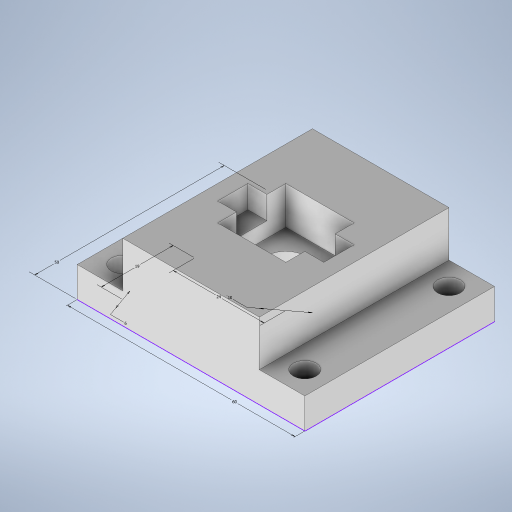
# Autodesk Inventor part: Bartosz_Zukowski_model_nr_7
Saved by Autodesk Inventor 2024 (Build 280153000, 153)
## iProperties
Created: 2024-03-20
Part Number: Bartosz_Zukowski_model_nr_7
Material: Ogólny
Document SubType Name: Modeling
Designer: student156p
Density: 1 g/cm^3
Appearance: Domyślna
Author: student156p
Autodesk Inventor part; units mm, degrees
ref_plane "YZ Plane" through (0, 0, 0) normal (1, 0, 0) x (0, 1, 0)
ref_plane "XZ Plane" through (0, 0, 0) normal (0, 1, 0) x (-1, 0, 0)
ref_plane "XY Plane" through (0, 0, 0) normal (0, 0, 1) x (1, 0, 0)
sketch "podstawa" plane through (0, 0, 0) normal (0, 0, 1) x (1, 0, 0)
  line L0 (-30, -25) -> (30, -25)
  line L1 (30, -25) -> (30, 25)
  line L2 (30, 25) -> (-30, 25)
  line L3 (-30, 25) -> (-30, -25)
  circle A0 centre (0, 0) radius 5
  line L4 (0, 0) -> (24, 0) construction
  line L5 (24, 0) -> (24, 19) construction
  circle A1 centre (24, 19) radius 3
  line L6 (0, 25) -> (0, -25) construction
  circle A2 centre (-24, 19) radius 3
  line L7 (-30, 0) -> (30, 0) construction
  circle A3 centre (24, -19) radius 3
  circle A4 centre (-24, -19) radius 3
  dimension "d0" = 60
  dimension "d1" = 50
  dimension "d9" = 10
  dimension "d26" = 24
  dimension "d27" = 19
  dimension "d28" = 6
  constraints: 16 end point, 5 centre point, 4 midpoint, 3 symmetric about line, 2 coincident, 2 horizontal, 2 parallel, 2 perpendicular, 3 other
  measures "d0" distance of L1.end L2.end
  measures "d1" distance of L0.end L1.end
  measures "d9" diameter of A0
  measures "d26" distance of L4.start L4.end
  measures "d27" distance of L4.end L5.end
  measures "d28" diameter of A1
extrude "Wyciągnięcie proste1" add sketch "podstawa" along normal blind 8 contours L3 L2 L1 L0 | A1 | A2 | A3 | A4
sketch "nakladka" plane through (0, 0, 8) normal (0, 0, 1) x (1, 0, 0)
  line L0 (18, -25) -> (-18, -25)
  line L1 (-18, -25) -> (-18, 25)
  line L2 (-18, 25) -> (18, 25)
  line L3 (18, 25) -> (18, -25)
  line L4 (18, -25) -> (-18, 25) construction
  line L5 (-18, -25) -> (18, 25) construction
  line L6 (-9, -9) -> (9, -9)
  line L7 (9, -9) -> (9, 9)
  line L8 (9, 9) -> (-9, 9)
  line L9 (-9, 9) -> (-9, -9)
  line L10 (-9, -9) -> (9, 9) construction
  line L11 (9, -9) -> (-9, 9) construction
  point P0 (0, 0)
  dimension "d12" = 36
  dimension "d13" = 50
  dimension "d14" = 18
  dimension "d15" = 18
  constraints: 24 end point, 4 midpoint, 4 parallel, 2 horizontal, 2 perpendicular
  measures "d12" distance of L1.end L2.end
  measures "d13" distance of L2.end L0.start
  measures "d14" distance of L7.end L8.end
  measures "d15" distance of L6.end L7.end
extrude "Wyciągnięcie proste2" add sketch "nakladka" along normal blind 12
sketch "srodek_2mm" plane through (0, 0, 8) normal (0, 0, 1) x (1, 0, 0)
  line L0 (-9, -9) -> (9, -9)
  line L1 (9, -9) -> (9, 9)
  line L2 (9, 9) -> (-9, 9)
  line L3 (-9, 9) -> (-9, -9)
  line L4 (-9, -9) -> (9, 9) construction
  line L5 (9, -9) -> (-9, 9) construction
  circle A0 centre (0, 0) radius 5
  constraints: 12 end point, 2 midpoint, 2 parallel, 1 centre point, 1 coincident, 1 horizontal, 1 perpendicular
extrude "Wyciągnięcie proste3" add sketch "srodek_2mm" along normal blind 2
sketch "wyciecie_gora_6mm" plane through (0, 0, 20) normal (0, 0, 1) x (1, 0, 0)
  line L0 (-14, -4) -> (14, -4)
  line L1 (14, -4) -> (14, 4)
  line L2 (14, 4) -> (-14, 4)
  line L3 (-14, 4) -> (-14, -4)
  line L4 (-14, -4) -> (14, 4) construction
  line L5 (14, -4) -> (-14, 4) construction
  point P0 (0, 0)
  dimension "d20" = 28
  dimension "d21" = 8
  constraints: 12 end point, 2 midpoint, 2 parallel, 1 horizontal, 1 perpendicular
  measures "d20" distance of L1.end L2.end
  measures "d21" distance of L0.end L1.end
extrude "Wyciągnięcie proste4" cut sketch "wyciecie_gora_6mm" against normal blind 6
extrude "Wyciągnięcie proste5" cut sketch "podstawa" along normal through all contours A1 | A2 | A3 | A4
